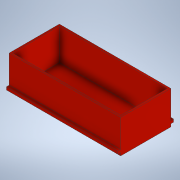
# Autodesk Inventor part: caja de mascarilllas
Saved by Autodesk Inventor 2021.1 (Build 251245000, 245)
## iProperties
Created: 2021-01-01
Part Number: caja de mascarilllas
Material: Generic
Document SubType Name: Modeling
Designer: Bolisteward
Density: 1 g/cm^3
Appearance: Default
Author: Bolisteward
Autodesk Inventor part; units mm, degrees
ref_plane "YZ Plane" through (0, 0, 0) normal (1, 0, 0) x (0, 1, 0)
ref_plane "XZ Plane" through (0, 0, 0) normal (0, 1, 0) x (-1, 0, 0)
ref_plane "XY Plane" through (0, 0, 0) normal (0, 0, 1) x (1, 0, 0)
sketch "Sketch1" plane through (0, 0, 0) normal (0, 1, 0) x (-1, 0, 0)
  line L0 (0, 0) -> (200, 0)
  line L1 (200, 0) -> (200, -90)
  line L2 (200, -90) -> (0, -90)
  line L3 (0, -90) -> (0, 0)
  line L4 (197, -87) -> (197, -3)
  line L5 (197, -3) -> (3, -3)
  line L6 (3, -3) -> (3, -87)
  line L7 (3, -87) -> (197, -87)
  dimension "d0" = 200
  dimension "d1" = 90
  dimension "d2" = 3
  constraints: 16 end point, 4 parallel, 2 perpendicular, 1 horizontal, 3 other
  measures "d0" distance of L1.end L2.end
  measures "d1" distance of L0.end L1.end
  measures "d2" distance between parallel lines of L1 L4
extrude "Extrusion1" add sketch "Sketch1" along normal blind 60
sketch "Sketch2" plane through (-200, 0, 0) normal (0, 0, 1) x (1, 0, 0)
  line L0 (0, 0) -> (0, 60) projected
  line L1 (200, 0) -> (200, 60) projected
  line L2 (0, 10) -> (200, 10)
  line L3 (200, 10) -> (200, 5)
  line L4 (200, 5) -> (0, 5)
  line L5 (0, 5) -> (0, 10)
  line L6 (0, 0) -> (200, 0) projected
  point P0 (0, 5)
  dimension "d5" = 5
  dimension "d6" = 5
  constraints: 8 end point, 2 parallel, 2 point on line, 1 horizontal, 1 perpendicular
  measures "d5" distance of L2.end L3.end
  measures "d6" distance between parallel lines of L6 L4
extrude "Extrusion2" add sketch "Sketch2" along normal blind 5 contours L0 L2 L1 L4
sketch "Sketch3" plane through (0, 0, -90) normal (0, 0, -1) x (-1, 0, 0)
  line L0 (0, 0) -> (0, 60) projected
  line L1 (200, 0) -> (200, 60) projected
  line L2 (0, 10) -> (200, 10)
  line L3 (200, 10) -> (200, 5)
  line L4 (200, 5) -> (0, 5)
  line L5 (0, 5) -> (0, 10)
  line L6 (0, 0) -> (200, 0) projected
  point P0 (0, 5)
  dimension "d9" = 5
  dimension "d10" = 5
  constraints: 8 end point, 2 parallel, 2 point on line, 1 horizontal, 1 perpendicular
  measures "d9" distance of L2.end L3.end
  measures "d10" distance between parallel lines of L6 L4
extrude "Extrusion3" add sketch "Sketch3" along normal blind 5 contours L0 L2 L1 L4
sketch "Sketch4" plane through (0, 0, 0) normal (0, -1, 0) x (1, 0, 0)
  line L0 (-197, -3) -> (-197, -87) projected
  line L1 (-3, -3) -> (-197, -3)
  line L2 (-197, -3) -> (-197, -87)
  line L3 (-197, -87) -> (-3, -87)
  line L4 (-3, -87) -> (-3, -3)
  line L5 (-50, -30) -> (-150, -30)
  line L6 (-150, -30) -> (-150, -60)
  line L7 (-150, -60) -> (-50, -60)
  line L8 (-50, -60) -> (-50, -30)
  line L9 (-200, -90) -> (-200, 0) projected
  line L10 (-200, 0) -> (0, 0) projected
  dimension "d13" = 100
  dimension "d14" = 30
  dimension "d16" = 50
  dimension "d17" = 30
  constraints: 16 end point, 4 parallel, 2 horizontal, 2 perpendicular
  measures "d13" distance of L7.end L6.end
  measures "d14" distance of L6.end L5.end
  measures "d16" distance between parallel lines of L6 L9
  measures "d17" distance between parallel lines of L5 L10
extrude "Extrusion4" add sketch "Sketch4" against normal blind 3
body "Solid1"
